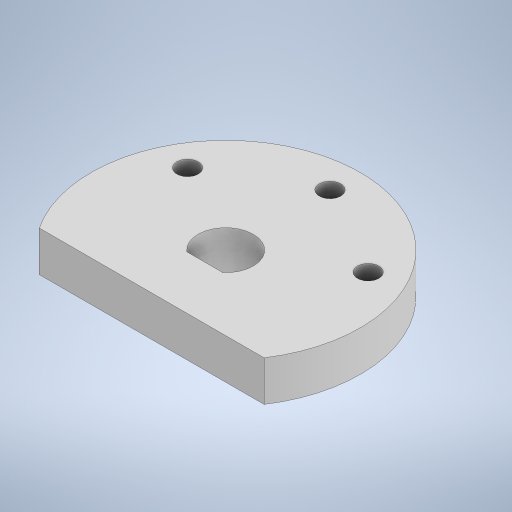
# Autodesk Inventor part: 射出_留め具2
Saved by Autodesk Inventor 2023 (Build 270158000, 158)
## iProperties
Created: 2022-05-04
Part Number: 射出_留め具2
Material: 一般
Document SubType Name: Modeling
Designer: yuta
Density: 1 g/cm^3
Appearance: 既定
Author: yuta
Autodesk Inventor part; units mm, degrees
ref_plane "YZ Plane" through (0, 0, 0) normal (1, 0, 0) x (0, 1, 0)
ref_plane "XZ Plane" through (0, 0, 0) normal (0, 1, 0) x (-1, 0, 0)
ref_plane "XY Plane" through (0, 0, 0) normal (0, 0, 1) x (1, 0, 0)
sketch "スケッチ1" plane through (0, 0, 0) normal (0, 1, 0) x (-1, 0, 0)
  arc A0 (-16.7033, 11) -> (16.7033, 11) centre (0, 0) ccw
  line L0 (16.7033, 11) -> (-16.7033, 11)
  point P0 (0, 11)
  dimension "d0" = 40
  dimension "d1" = 11
  constraints: 2 end point, 2 point on circle, 1 centre point, 1 coincident, 1 horizontal
  measures "d0" diameter of A0
  measures "d1" distance of point (0, 0) point (0, 11)
extrude "押し出し1" add sketch "スケッチ1" along normal blind 6
sketch "スケッチ3" plane through (0, 6, 0) normal (0, 1, 0) x (1, 0, 0)
  arc A0 (2.6833, -3.1) -> (-2.6833, -3.1) centre (0, 0) ccw
  line L0 (-2.6833, -3.1) -> (2.6833, -3.1)
  point P0 (0, -3.1)
  dimension "d12" = 8.2
  dimension "d13" = 3.1
  constraints: 2 end point, 2 point on circle, 1 centre point, 1 coincident, 1 horizontal
  measures "d12" diameter of A0
  measures "d13" distance of point (0, 0) point (0, -3.1)
extrude "押し出し2" cut sketch "スケッチ3" against normal blind 6
sketch "スケッチ4" plane through (0, 6, 0) normal (0, 1, 0) x (1, 0, 0)
  circle A0 centre (0, 0) radius 15.5 construction
  line L0 (0, 0) -> (-19.4826, 11.2483) construction
  line L1 (0, 0) -> (29.419, 16.9851) construction
  line L2 (0, 0) -> (0, 25.14) construction
  point P0 (0, 15.5)
  point P1 (-13.4234, 7.75)
  point P2 (-13.4234, 7.75)
  point P3 (0, 15.5)
  point P4 (13.4234, 7.75)
  dimension "d16" = 31
  dimension "d17" = 60
  dimension "d18" = 60
  constraints: 6 end point, 3 coincident, 3 point on circle, 2 point on line, 1 centre point, 1 vertical
  measures "d16" diameter of A0
  measures "d17" angle of L0 L2
  measures "d18" angle of L2 L1
hole "穴2" at (0, 6, -15.5) at (-13.4234, 6, -7.75) at (13.4234, 6, -7.75) direction (0, -1, 0) diameter 3.2 end through all
